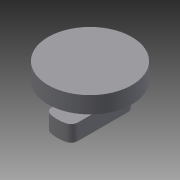
# Autodesk Inventor part: EarConnector
Saved by Autodesk Inventor 2014 SP1 (Build 180222100, 222)
## iProperties
Created: 2013-10-30
Part Number: EarConnector
Material: Generic
Document SubType Name: Modeling
Designer: david
Density: 1 g/cm^3
Appearance: Default
Author: david
Autodesk Inventor part; units mm, degrees
ref_plane "YZ Plane" through (0, 0, 0) normal (1, 0, 0) x (0, 1, 0)
ref_plane "XZ Plane" through (0, 0, 0) normal (0, 1, 0) x (-1, 0, 0)
ref_plane "XY Plane" through (0, 0, 0) normal (0, 0, 1) x (1, 0, 0)
sketch "Sketch1" plane through (0, 0, 0) normal (0, 1, 0) x (-1, 0, 0)
  circle A0 centre (0, 0) radius 12.5
  dimension "d0" = 25
  constraints: 1 centre point, 1 coincident
  measures "d0" diameter of A0
extrude "Extrusion1" add sketch "Sketch1" along normal blind 5
sketch "Sketch2" plane through (0, 0, 0) normal (0, -1, 0) x (1, 0, 0)
  circle A0 centre (0, 0) radius 12.5 projected
  circle A1 centre (0, 0) radius 3.9
  dimension "d3" = 7.8
  constraints: 1 centre point, 1 coincident
  measures "d3" diameter of A1
extrude "Extrusion2" add sketch "Sketch2" along normal blind 5.2 contours A1
sketch "Sketch3" plane through (0, -5.2, 0) normal (0, -1, 0) x (1, 0, 0)
  circle A0 centre (0, 0) radius 3.9 projected
  line L0 (-3.9, 8.9906) -> (-3.9, -8.9906)
  line L1 (3.9, 8.9906) -> (3.9, -8.9906)
  line L2 (0, 15.7328) -> (0, -15.032) construction
  circle A1 centre (0, 0) radius 12.5 construction
  arc A2 (-5, 11.4564) -> (-5, -11.4564) centre (0, 0) ccw construction
  arc A3 (5, -11.4564) -> (5, 11.4564) centre (0, 0) ccw construction
  arc A4 (3.9, 8.9906) -> (-3.9, 8.9906) centre (0, 0) ccw
  arc A5 (-3.9, -8.9906) -> (3.9, -8.9906) centre (0, 0) ccw
  dimension "d13" = 9.8
  dimension "d19" = 9.8
  constraints: 12 point on circle, 6 end point, 4 centre point, 2 coincident, 2 parallel, 2 tangent, 1 concentric, 1 vertical
  measures "d13" radius of A4
  measures "d19" radius of A5
extrude "Extrusion3" add sketch "Sketch3" along normal blind 4.8
fillet "Fillet2" radius 2 4 edges at (-3.9, -7.6, 8.9906) (3.9, -7.6, 8.9906) (-3.9, -7.6, -8.9906) (3.9, -7.6, -8.9906)
equation "\"d0\" = HeadConnectorOuterSize"
equation "\"d3\" = HeadConnectorWidth - HeadConnectorTolerance"
equation "\"d4\" = HeadConnectorOuterHeight + HeadConnectorTolerance"
equation "\"d13\" = 0.5 * HeadConnectorDiam - HeadConnectorTolerance"
equation "\"d19\" = 0.5 * HeadConnectorDiam - HeadConnectorTolerance"
equation "\"d10\" = HeadConnectorHeight - HeadConnectorTolerance"
equation "\"HeadConnectorOuterSize\" = 25"
equation "\"HeadConnectorWidth\" = 8"
equation "\"HeadConnectorTolerance\" = 0.2"
equation "\"HeadConnectorOuterHeight\" = 5"
equation "\"HeadConnectorDiam\" = 20"
equation "\"HeadConnectorHeight\" = 5"
body "Solid1"
